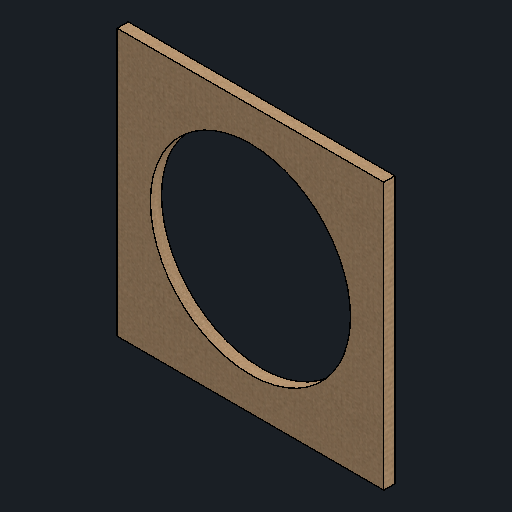
# Autodesk Inventor part: Part1
Saved by Autodesk Inventor 2026.2 (Build 302298000, 298)
## iProperties
Created: 2026-06-15
Part Number: Part1
Material: MDF Medium Density Fiberboard
Document SubType Name: Modeling
Designer: JoshuaEah
Density: 0.8 g/cm^3
Appearance: Cardboard - Corrugated
Author: JoshuaEah
Autodesk Inventor part; units mm, degrees
ref_plane "YZ Plane" through (0, 0, 0) normal (1, 0, 0) x (0, 1, 0)
ref_plane "XZ Plane" through (0, 0, 0) normal (0, 1, 0) x (-1, 0, 0)
ref_plane "XY Plane" through (0, 0, 0) normal (0, 0, 1) x (1, 0, 0)
sketch "Sketch1" plane through (0, 0, 0) normal (0, 0, 1) x (1, 0, 0)
  line L0 (0, 0) -> (304.8, 0)
  line L1 (304.8, 0) -> (304.8, 304.8)
  line L2 (304.8, 304.8) -> (0, 304.8)
  line L3 (0, 304.8) -> (0, 0)
  circle A0 centre (152.4, 152.4) radius 114.3
  point P0 (304.8, 152.4)
  point P1 (152.4, 304.8)
  dimension "d0" = 304.8
  dimension "d1" = 228.6
  constraints: 8 end point, 2 midpoint, 2 parallel, 2 perpendicular, 1 centre point, 1 coincident, 1 horizontal, 1 horizontal alignment, 1 vertical alignment
  measures "d0" distance of L1.end L2.end
  measures "d1" diameter of A0
extrude "Extrusion1" add sketch "Sketch1" along normal blind 12.7
body "Solid1"
